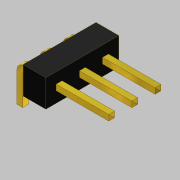
# Autodesk Inventor part: 3 Pin Header 90 Degree
Saved by Autodesk Inventor 2012 (Build 160160000, 160)
## iProperties
Category: FIRST
Manager: Ed Sparks
Company: FirstCadLibrary
Shininess: 64.0
Length Units: 11269
Angle Units: 11279
Time Units: 11290
Mass Units: 11283
Length Display Precision: 3
Angle Display Precision: 2
Compacted: True
Part Number: 3 Pin Header 90 Degree
Document SubType Name: Modeling
Created: 2007-12-18
Material: ABS Plastic
Catalog Web Link: www.firstcadlibrary.com
Designer: Ed Sparks
Engineer: Ed Sparks
Density: 1.06 g/cm^3
Mass: 0.0776984 g
Surface Area: 1.86142 cm^2
Volume: 0.0733004 cm^3
Density: 0.0
Volumn: 0.0
Area: 0.0
PropertySet Name: Model Information
Control State: 0
Master: False
Checked Out: False
Author: Ed Sparks
Keywords: FIRST
Autodesk Inventor part; units mm, degrees
ref_plane "YZ Plane" through (0, 0, 0) normal (1, 0, 0) x (0, 1, 0)
ref_plane "XZ Plane" through (0, 0, 0) normal (0, 1, 0) x (-1, 0, 0)
sketch "Sketch1" plane through (0, 0, 0) normal (0, 0, 1) x (1, 0, 0)
  line L0 (-0.3175, 0.3175) -> (0.3175, 0.3175)
  line L1 (0.3175, 0.3175) -> (0.3175, -0.3175)
  line L2 (0.3175, -0.3175) -> (-0.3175, -0.3175)
  line L3 (-0.3175, -0.3175) -> (-0.3175, 0.3175)
  line L4 (2.2225, 0.3175) -> (2.8575, 0.3175)
  line L5 (2.8575, 0.3175) -> (2.8575, -0.3175)
  line L6 (2.8575, -0.3175) -> (2.2225, -0.3175)
  line L7 (2.2225, -0.3175) -> (2.2225, 0.3175)
  line L8 (-2.8575, 0.3175) -> (-2.2225, 0.3175)
  line L9 (-2.2225, 0.3175) -> (-2.2225, -0.3175)
  line L10 (-2.2225, -0.3175) -> (-2.8575, -0.3175)
  line L11 (-2.8575, -0.3175) -> (-2.8575, 0.3175)
  line L12 (0, 0) -> (0, 0.3175) construction
  line L13 (0, 0) -> (0, -0.3175) construction
  line L14 (0, 0) -> (0.3175, 0) construction
  line L15 (0, 0) -> (-0.3175, 0) construction
  dimension "d0" = 0.635
  dimension "d1" = 2.54
  dimension "d2" = 2.54
  constraints: 32 end point, 7 equal length, 6 parallel, 4 midpoint, 3 horizontal, 3 perpendicular, 2 collinear, 1 other
  measures "d0" distance of L0.start L0.end
  measures "d1" distance of L5.end L1.end
  measures "d2" distance of L9.end L1.end
sketch "Sketch2" plane through (0, 0, 0) normal (1, 0, 0) x (0, 1, 0)
  line L0 (0, 0) -> (-0.3175, 0) projected
  line L1 (0, 0) -> (0.3175, 0) projected
  line L2 (0, 0) -> (0, 3.5)
  line L3 (-0.5, 4) -> (-10, 4)
  arc A0 (0, 3.5) -> (-0.5, 4) centre (-0.5, 3.5) ccw
  point P0 (0, 0)
  point P1 (0, 0)
  point P2 (0, 4)
  dimension "d3" = 4
  dimension "d4" = 10
  dimension "d5" = 0.5
  constraints: 4 end point, 2 point on circle, 2 point on line, 2 tangent, 1 centre point, 1 horizontal, 1 vertical
  measures "d3" distance of L2.start point (0, 4)
  measures "d4" distance of point (0, 4) L3.end
  measures "d5" radius of A0
sweep "Sweep1" add profiles "Sketch1" path "Sketch2" path curves L2 A0 L3
ref_plane "Work Plane1" through (2.2225, -4, 3.6825) normal (0, -1, 0) x (1, 0, 0)
sketch "Sketch3" plane through (2.2225, -4, 3.6825) normal (0, -1, 0) x (1, 0, 0)
  line L0 (-6.2225, 1.8175) -> (1.7775, 1.8175)
  line L1 (1.7775, 1.8175) -> (1.7775, -1.1825)
  line L2 (1.7775, -1.1825) -> (-6.2225, -1.1825)
  line L3 (-6.2225, -1.1825) -> (-6.2225, 1.8175)
  line L4 (-2.54, 0.635) -> (-1.905, 0.635) projected
  line L5 (-1.905, 0.635) -> (-1.905, 0) projected
  line L6 (-1.905, 0) -> (-2.54, 0) projected
  line L7 (-2.54, 0) -> (-2.54, 0.635) projected
  line L8 (-1.905, 0.635) -> (1.7775, 1.8175) construction
  line L9 (-2.54, 0.635) -> (-6.2225, 1.8175) construction
  line L10 (-2.54, 0) -> (-6.2225, -1.1825) construction
  line L11 (-1.905, 0) -> (1.7775, -1.1825) construction
  dimension "d8" = 8
  dimension "d9" = 3
  constraints: 16 end point, 3 equal length, 2 parallel, 1 horizontal, 1 perpendicular
  measures "d8" distance of L0.start L0.end
  measures "d9" distance of L0.end L1.end
extrude "Extrusion1" add sketch "Sketch3" against normal blind 2.5
chamfer "Chamfer1" distance 0.25 angle 45 24 edges at (2.54, -10, 4.3175) (2.8575, -10, 4) (2.54, -10, 3.6825) (2.2225, -10, 4) (0.3175, -10, 4) (0, -10, 4.3175) (-0.3175, -10, 4) (0, -10, 3.6825) (-2.2225, -10, 4) (-2.54, -10, 4.3175) (-2.8575, -10, 4) (-2.54, -10, 3.6825) (2.8575, 0, 0) (2.54, -0.3175, 0) (2.2225, 0, 0) (2.54, 0.3175, 0) (0, 0.3175, 0) (0, -0.3175, 0) (0.3175, 0, 0) (-0.3175, 0, 0) (-2.2225, 0, 0) (-2.54, 0.3175, 0) (-2.8575, 0, 0) (-2.54, -0.3175, 0)
body "Solid1"
